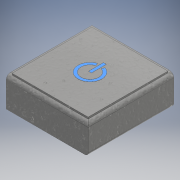
# Autodesk Inventor part: PRZYCISK IO
Saved by Autodesk Inventor 2017 SP1 (Build 210196100, 196)
## iProperties
Created: 2021-03-07
Part Number: PRZYCISK IO
Material: Tworzywo sztuczne, nieprzezroczyste czarne
Document SubType Name: Modeling
Designer: Administrator
Density: 0.952 g/cm^3
Appearance: Teksturowany - szary
Author: Administrator
Autodesk Inventor part; units mm, degrees
ref_plane "YZ Plane" through (0, 0, 0) normal (1, 0, 0) x (0, 1, 0)
ref_plane "XZ Plane" through (0, 0, 0) normal (0, 1, 0) x (-1, 0, 0)
ref_plane "XY Plane" through (0, 0, 0) normal (0, 0, 1) x (1, 0, 0)
sketch "Szkic1" plane through (0, 0, 0) normal (0, 0, 1) x (1, 0, 0)
  line L0 (206.45, -143.65) -> (206.45, -129.275)
  line L1 (206.45, -129.275) -> (220.2, -129.275)
  line L2 (206.45, -143.65) -> (220.2, -143.65)
  line L3 (220.2, -129.275) -> (220.2, -143.65)
  constraints: 8 end point
extrude "Wyciągnięcie proste1" add sketch "Szkic1" against normal blind 5.2
fillet "Zaokrąglenie1" radius 0.5 1 edges at (220.2, -136.4625, -5.2)
sketch "Szkic2" plane through (0, 0, 0) normal (0, 0, 1) x (1, 0, 0)
  line L0 (206.95, -129.775) -> (219.7, -129.775)
  line L1 (219.7, -129.775) -> (219.7, -143.15)
  line L2 (219.7, -143.15) -> (206.95, -143.15)
  line L3 (206.95, -143.15) -> (206.95, -129.775)
  line L4 (206.45, -129.275) -> (220.2, -129.275) projected
  line L5 (220.2, -129.275) -> (220.2, -143.65) projected
  line L6 (206.45, -129.275) -> (220.2, -129.275)
  line L7 (220.2, -129.275) -> (220.2, -143.65)
  line L8 (220.2, -143.65) -> (206.45, -143.65)
  line L9 (206.45, -143.65) -> (206.45, -129.275)
  point P0 (0, 0)
  constraints: 16 end point, 4 parallel, 2 horizontal, 2 perpendicular
extrude "Wyciągnięcie proste2" cut sketch "Szkic2" against normal blind 0.25
sketch "Szkic3" plane through (0, 0, 0) normal (0, 0, 1) x (1, 0, 0)
  line L0 (213.075, -133.9625) -> (213.575, -133.9625)
  line L1 (213.575, -133.9625) -> (213.575, -136.4625)
  line L2 (213.575, -136.4625) -> (213.075, -136.4625)
  line L3 (213.075, -136.4625) -> (213.075, -133.9625)
  line L4 (212.875, -134.9835) -> (212.875, -135.0316)
  line L5 (212.875, -135.0316) -> (212.7039, -134.5614)
  line L6 (213.775, -135.0316) -> (213.9461, -134.5614)
  arc A0 (212.7039, -134.5614) -> (213.9461, -134.5614) centre (213.325, -136.4625) ccw
  arc A1 (212.875, -135.0316) -> (213.775, -135.0316) centre (213.325, -136.4625) ccw
  point P0 (0, 0)
  constraints: 14 end point, 4 point on circle, 2 centre point, 2 parallel, 1 horizontal, 1 perpendicular
extrude "Wyciągnięcie proste3" cut sketch "Szkic3" against normal blind 0.5
sketch "Szkic4" plane through (0, 0, -0.5) normal (0, 0, 1) x (1, 0, 0)
  line L0 (213.075, -133.9625) -> (213.575, -133.9625) projected
  line L1 (213.075, -136.4625) -> (213.075, -133.9625) projected
  line L2 (213.575, -136.4625) -> (213.075, -136.4625) projected
  line L3 (213.575, -133.9625) -> (213.575, -136.4625) projected
  line L4 (212.7039, -134.5614) -> (212.875, -135.0316) projected
  arc A0 (212.7039, -134.5614) -> (213.9461, -134.5614) centre (213.325, -136.4625) ccw projected
  line L5 (213.775, -135.0316) -> (213.9461, -134.5614) projected
  arc A1 (212.875, -135.0316) -> (213.775, -135.0316) centre (213.325, -136.4625) ccw projected
  point P0 (0, 0)
extrude "Wyciągnięcie proste4" add sketch "Szkic4" along normal blind 0.51
fillet "Zaokrąglenie2" radius 0.75 2 edges at (220.2, -136.4625, -0.25) (213.325, -143.65, -0.25)
